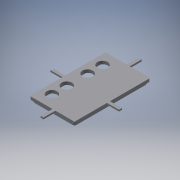
# Autodesk Inventor part: iceTubeClockTop
Saved by Autodesk Inventor 2016 (Build 200138000, 138)
## iProperties
Created: 2016-04-01
Part Number: iceTubeClockTop
Material: Generic
Document SubType Name: Modeling
Designer: boztalay
Density: 1 g/cm^3
Appearance: Default
Author: boztalay
Autodesk Inventor part; units mm, degrees
ref_plane "YZ Plane" through (0, 0, 0) normal (1, 0, 0) x (0, 1, 0)
ref_plane "XZ Plane" through (0, 0, 0) normal (0, 1, 0) x (-1, 0, 0)
ref_plane "XY Plane" through (0, 0, 0) normal (0, 0, 1) x (1, 0, 0)
sketch "Sketch1" plane through (0, 0, 0) normal (0, 1, 0) x (-1, 0, 0)
  line L0 (-47.625, 80.645) -> (47.625, 80.645)
  line L1 (47.625, 80.645) -> (47.625, -80.645)
  line L2 (47.625, -80.645) -> (-47.625, -80.645)
  line L3 (-47.625, -80.645) -> (-47.625, 80.645)
  line L4 (-47.625, 80.645) -> (47.625, -80.645) construction
  line L5 (47.625, 80.645) -> (-47.625, -80.645) construction
  point P0 (0, 0)
  dimension "d0" = 161.29
  dimension "d1" = 95.25
  constraints: 12 end point, 2 midpoint, 2 parallel, 1 horizontal, 1 perpendicular
  measures "d0" distance of L0.end L1.end
  measures "d1" distance of L1.end L2.end
extrude "Extrusion1" add sketch "Sketch1" along normal blind 6.35
sketch "Sketch3" plane through (0, 0, 0) normal (0, -1, 0) x (1, 0, 0)
  line L0 (-44.45, 77.47) -> (44.45, 77.47)
  line L1 (44.45, 77.47) -> (44.45, -77.47)
  line L2 (44.45, -77.47) -> (-44.45, -77.47)
  line L3 (-44.45, -77.47) -> (-44.45, 77.47)
  line L4 (-44.45, 77.47) -> (44.45, -77.47) construction
  line L5 (44.45, 77.47) -> (-44.45, -77.47) construction
  line L6 (-41.275, 74.295) -> (41.275, 74.295)
  line L7 (41.275, 74.295) -> (41.275, -74.295)
  line L8 (41.275, -74.295) -> (-41.275, -74.295)
  line L9 (-41.275, -74.295) -> (-41.275, 74.295)
  line L10 (-41.275, 74.295) -> (41.275, -74.295) construction
  line L11 (41.275, 74.295) -> (-41.275, -74.295) construction
  point P0 (0, 0)
  dimension "d4" = 154.94
  dimension "d5" = 88.9
  dimension "d6" = 148.59
  dimension "d7" = 82.55
  constraints: 24 end point, 4 midpoint, 4 parallel, 2 horizontal, 2 perpendicular
  measures "d4" distance of L0.end L1.end
  measures "d5" distance of L1.end L2.end
  measures "d6" distance of L6.end L7.end
  measures "d7" distance of L7.end L8.end
extrude "Extrusion2" add sketch "Sketch3" along normal blind 4.7625
sketch "Sketch4" plane through (0, 6.35, 0) normal (0, 1, 0) x (1, 0, 0)
  line L0 (24.765, -53.975) -> (-24.765, -53.975) construction
  line L1 (-24.765, -53.975) -> (-24.765, 53.975) construction
  line L2 (-24.765, 53.975) -> (24.765, 53.975) construction
  line L3 (24.765, 53.975) -> (24.765, -53.975) construction
  line L4 (24.765, -53.975) -> (-24.765, 53.975) construction
  line L5 (-24.765, -53.975) -> (24.765, 53.975) construction
  circle A0 centre (-24.765, -53.975) radius 10.9982
  circle A1 centre (-24.765, 53.975) radius 10.9982
  circle A2 centre (-24.765, -22.225) radius 10.9982
  circle A3 centre (-24.765, 22.225) radius 10.9982
  line L6 (47.625, -80.645) -> (47.625, 80.645) projected
  point P0 (0, 0)
  dimension "d12" = 21.9964
  dimension "d13" = 21.9964
  dimension "d15" = 21.9964
  dimension "d17" = 31.75
  dimension "d18" = 21.9964
  dimension "d19" = 31.75
  dimension "d25" = 44.45
  dimension "d26" = 72.39
  constraints: 12 end point, 4 centre point, 2 coincident, 2 midpoint, 2 parallel, 2 point on line, 1 horizontal, 1 perpendicular
  measures "d12" diameter of A0
  measures "d13" diameter of A1
  measures "d15" diameter of A2
  measures "d17" distance of A2.centre L0.end
  measures "d18" diameter of A3
  measures "d19" distance of L1.end A3.centre
  measures "d25" distance of A3.centre A2.centre
  measures "d26" distance between parallel lines of L6 L1
extrude "Extrusion3" cut sketch "Sketch4" against normal up to next
fillet "Fillet1" radius 3.175 12 edges at (47.625, 3.175, 80.645) (-47.625, 3.175, 80.645) (47.625, 3.175, -80.645) (-47.625, 3.175, -80.645) (44.45, -2.3813, -77.47) (44.45, -2.3813, 77.47) (-44.45, -2.3813, -77.47) (-41.275, -2.3813, 74.295) (-44.45, -2.3813, 77.47) (41.275, -2.3813, 74.295) (41.275, -2.3813, -74.295) (-41.275, -2.3813, -74.295)
sketch "Sketch5" plane through (44.45, 0, -80.645) normal (0, 0, -1) x (-1, 0, 0)
  line L0 (88.9, 6.35) -> (0, 6.35) projected
  line L1 (40.1232, 6.35) -> (46.4732, 6.35)
  line L2 (46.4732, 6.35) -> (46.4732, 2.8141)
  line L3 (46.4732, 2.8141) -> (40.1232, 2.8141)
  line L4 (40.1232, 2.8141) -> (40.1232, 6.35)
  point P0 (44.45, 0)
  dimension "d37" = 6.35
  constraints: 8 end point, 2 parallel, 1 horizontal, 1 perpendicular, 1 point on line
  measures "d37" distance of L2.end L3.end
sketch "Sketch6" plane through (-47.625, 0, -77.47) normal (-1, 0, 0) x (0, 0, 1)
  line L0 (0, 6.35) -> (154.94, 6.35) projected
  line L1 (88.6968, 6.35) -> (88.6968, 0) projected
  line L2 (82.3468, 6.35) -> (88.6968, 6.35)
  line L3 (88.6968, 6.35) -> (88.6968, 3.175)
  line L4 (88.6968, 3.175) -> (82.3468, 3.175)
  line L5 (82.3468, 3.175) -> (82.3468, 6.35)
  point P0 (77.47, 0)
  dimension "d38" = 6.35
  constraints: 8 end point, 2 parallel, 1 horizontal, 1 midpoint, 1 perpendicular, 1 point on line
  measures "d38" distance of L3.end L4.end
sketch "Sketch7" plane through (47.625, 0, 77.47) normal (1, 0, 0) x (0, 0, -1)
  line L0 (154.94, 6.35) -> (0, 6.35) projected
  line L1 (66.2432, 6.35) -> (66.2432, 0) projected
  line L2 (72.5932, 6.35) -> (66.2432, 6.35)
  line L3 (66.2432, 6.35) -> (66.2432, 3.175)
  line L4 (66.2432, 3.175) -> (72.5932, 3.175)
  line L5 (72.5932, 3.175) -> (72.5932, 6.35)
  point P0 (77.47, 0)
  dimension "d36" = 6.35
  constraints: 8 end point, 2 parallel, 1 horizontal, 1 midpoint, 1 perpendicular, 1 point on line
  measures "d36" distance of L3.end L4.end
sketch "Sketch8" plane through (-44.45, 0, 80.645) normal (0, 0, 1) x (1, 0, 0)
  line L0 (0, 6.35) -> (88.9, 6.35) projected
  line L1 (51.344, 6.35) -> (44.994, 6.35)
  line L2 (44.994, 6.35) -> (44.994, 2.9455)
  line L3 (44.994, 2.9455) -> (51.344, 2.9455)
  line L4 (51.344, 2.9455) -> (51.344, 6.35)
  point P0 (44.45, 0)
  dimension "d39" = 6.35
  constraints: 8 end point, 2 parallel, 1 horizontal, 1 perpendicular, 1 point on line
  measures "d39" distance of L2.end L3.end
extrude "Extrusion4" add sketch "Sketch8" along normal blind 25.4
extrude "Extrusion5" add sketch "Sketch5" along normal blind 25.4
extrude "Extrusion6" add sketch "Sketch6" along normal blind 25.4
extrude "Extrusion7" add sketch "Sketch7" along normal blind 25.4
body "Solid1"
